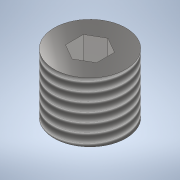
# Autodesk Inventor part: M6x6_DIN914
Saved by Autodesk Inventor 2020 (Build 240168000, 168)
## iProperties
Created: 2020-08-10
Part Number: M6x6_DIN914
Material: Steel, Mild
Document SubType Name: Modeling
Designer: Hesekiel
Density: 7.85 g/cm^3
Appearance: Semi-Polished
Mass: 1.1151 g
Surface Area: 1.71297 cm^2
Volume: 0.14205 cm^3
Author: Hesekiel
Autodesk Inventor part; units mm, degrees
ref_plane "YZ Plane" through (0, 0, 0) normal (1, 0, 0) x (0, 1, 0)
ref_plane "XZ Plane" through (0, 0, 0) normal (0, 1, 0) x (-1, 0, 0)
ref_plane "XY Plane" through (0, 0, 0) normal (0, 0, 1) x (1, 0, 0)
sketch "Sketch1" plane through (0, 0, 0) normal (0, 1, 0) x (-1, 0, 0)
  circle A0 centre (0, 0) radius 3
  dimension "d0" = 6
  constraints: 1 centre point, 1 coincident
  measures "d0" diameter of A0
extrude "Extrusion1" add sketch "Sketch1" along normal blind 6
sketch "Sketch2" plane through (0, 0, 0) normal (0, -1, 0) x (1, 0, 0)
  circle A0 centre (0, 0) radius 0.75
  circle A1 centre (0, 0) radius 3
  dimension "d3" = 1.5
  constraints: 2 centre point, 2 coincident
  measures "d3" diameter of A0
extrude "Extrusion2" cut sketch "Sketch2" against normal blind 1
loft "Loft1" add section 1 edges at (-0.75, 0, 0) section 2 edges at (3, 1, 0)
thread "Thread1" size "M6x0.75" class "6g" standard "ANSI Metric M Profile" full length
sketch "Sketch3" plane through (0, 6, 0) normal (0, 1, 0) x (1, 0, 0)
  line L0 (0, 0) -> (0, 1.5)
  line L1 (0, 1.5) -> (1.299, 0.75)
  line L2 (1.299, 0.75) -> (1.299, -0.75)
  line L3 (1.299, -0.75) -> (0, -1.5)
  line L4 (0, -1.5) -> (-1.299, -0.75)
  line L5 (-1.299, -0.75) -> (-1.299, 0.75)
  line L6 (-1.299, 0.75) -> (0, 1.5)
  dimension "d12" = 1.5
  constraints: 14 end point, 1 coincident, 1 vertical, 13 other
  measures "d12" distance of L0.start L0.end
extrude "Extrusion3" cut sketch "Sketch3" against normal blind 2
body "Solid1"
